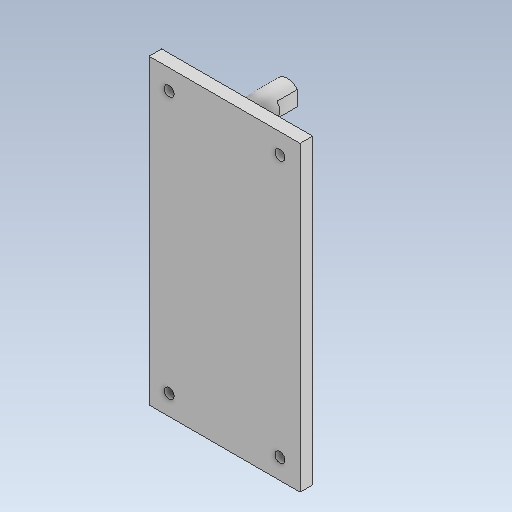
# Autodesk Inventor part: Gear_Platte_3D-Druck
Saved by Autodesk Inventor 2025.2 (Build 292293000, 293)
## iProperties
Created: 2025-02-25
Part Number: Gear_Platte_3D-Druck
Material: Generisch
Document SubType Name: Modeling
Designer: maria
Density: 1 g/cm^3
Appearance: Vorgabe
Author: maria
## iProperties of the stored document Gear_Platte_3D-Druck_3D-Druck.ipt
Created: 2025-02-25
Part Number: Gear_Platte_3D-Druck_3D-Druck
Material: Generisch
Document SubType Name: Modeling
Designer: maria
Density: 1 g/cm^3
Appearance: Vorgabe
Author: maria
Autodesk Inventor part; units mm, degrees
ref_plane "YZ Plane" through (0, 0, 0) normal (1, 0, 0) x (0, 1, 0)
ref_plane "XZ Plane" through (0, 0, 0) normal (0, 1, 0) x (-1, 0, 0)
ref_plane "XY Plane" through (0, 0, 0) normal (0, 0, 1) x (1, 0, 0)
sketch "Skizze1" plane through (0, 0, 0) normal (0, 1, 0) x (-1, 0, 0)
  line L0 (0, 0) -> (60, 0)
  line L1 (60, 0) -> (60, -120)
  line L2 (60, -120) -> (0, -120)
  line L3 (0, -120) -> (0, 0)
  dimension "d0" = 120
  dimension "d1" = 60
  constraints: 8 end point, 2 parallel, 1 horizontal, 1 perpendicular
  measures "d0" distance of L2.end L0.start
  measures "d1" distance of L0.start L0.end
extrude "Extrusion1" add sketch "Skizze1" along normal blind 5
sketch "Skizze2" plane through (0, 5, 0) normal (0, 1, 0) x (1, 0, 0)
  circle A0 centre (-30, 10) radius 4.9
  circle A1 centre (-30, 40) radius 4.9
  circle A2 centre (-30, 90) radius 4.9
  line L0 (-60, 0) -> (0, 0) projected
  line L1 (0, 0) -> (0, 120) projected
  dimension "d4" = 10
  dimension "d5" = 30
  dimension "d6" = 50
  dimension "d7" = 30
  dimension "d8" = 30
  dimension "d9" = 30
  dimension "d10" = 9.8
  dimension "d11" = 9.8
  dimension "d12" = 9.8
  constraints: 3 centre point
  measures "d4" distance from line of A0.centre L0
  measures "d5" distance of A1.centre A0.centre
  measures "d6" distance of A2.centre A1.centre
  measures "d7" distance from line of L1 A0.centre
  measures "d8" distance from line of L1 A1.centre
  measures "d9" distance from line of L1 A2.centre
  measures "d10" diameter of A0
  measures "d11" diameter of A1
  measures "d12" diameter of A2
extrude "Extrusion2" add sketch "Skizze2" along normal blind 20
sketch "Skizze3" plane through (0, 0, -120) normal (0, 0, -1) x (-1, 0, 0)
  line L0 (25.1, 5) -> (25.1, 25) projected
  line L1 (25.1, 6.7142) -> (25.1, 25)
  line L2 (34.9, 5) -> (34.9, 25) projected
  line L3 (34.9, 5) -> (34.9, 25)
  line L4 (60, 5) -> (0, 5) projected
  line L5 (23.3172, 25) -> (26.1, 25)
  line L6 (26.1, 25) -> (26.1, 17)
  line L7 (26.1, 17) -> (23.3172, 17)
  line L8 (23.3172, 17) -> (23.3172, 25)
  line L9 (36.4895, 25) -> (33.9, 25)
  line L10 (33.9, 25) -> (33.9, 17)
  line L11 (33.9, 17) -> (36.4895, 17)
  line L12 (36.4895, 17) -> (36.4895, 25)
  line L13 (34.9, 25) -> (25.1, 25) projected
  point P0 (0, 0)
  dimension "d19" = 8
  dimension "d20" = 1
  dimension "d21" = 1
  constraints: 20 end point, 6 point on line, 4 parallel, 2 horizontal, 2 perpendicular
  measures "d19" distance between parallel lines of L7 L13
  measures "d20" distance between parallel lines of L6 L0
  measures "d21" distance between parallel lines of L2 L10
extrude "Extrusion3" cut sketch "Skizze3" against normal blind 120 contours L7 L8 L5 L0 | L0 L5 L6 L7 | L11 L10 L9 L2 | L2 L9 L12 L11
sketch "Skizze4" plane through (0, 5, 0) normal (0, 1, 0) x (1, 0, 0)
  line L0 (0, 0) -> (0, 120) projected
  line L1 (-60, 0) -> (0, 0) projected
  line L2 (-60, 120) -> (-60, 0) projected
  line L3 (0, 120) -> (-60, 120) projected
  point P0 (-8, 8)
  point P1 (-52, 8)
  point P2 (-8, 112)
  point P3 (-52, 112)
  dimension "d31" = 8
  dimension "d32" = 8
  dimension "d33" = 8
  dimension "d34" = 8
  dimension "d35" = 8
  dimension "d36" = 8
  dimension "d37" = 8
  dimension "d38" = 8
  dimension "d39" = 104
  dimension "d40" = 44
  measures "d31" distance from line of point (-8, 8) L0
  measures "d32" distance from line of L1 point (-8, 8)
  measures "d33" distance from line of L1 point (-52, 8)
  measures "d34" distance from line of L2 point (-52, 8)
  measures "d35" distance from line of L2 point (-52, 112)
  measures "d36" distance from line of L3 point (-52, 112)
  measures "d37" distance from line of L3 point (-8, 112)
  measures "d38" distance from line of L0 point (-8, 112)
  measures "d39" distance of point (-52, 112) point (-52, 8)
  measures "d40" distance of point (-52, 112) point (-8, 112)
hole "Bohrung1" at (-8, 5, -8) at (-52, 5, -8) at (-8, 5, -112) at (-52, 5, -112) direction (0, -1, 0) diameter 4 depth 5
